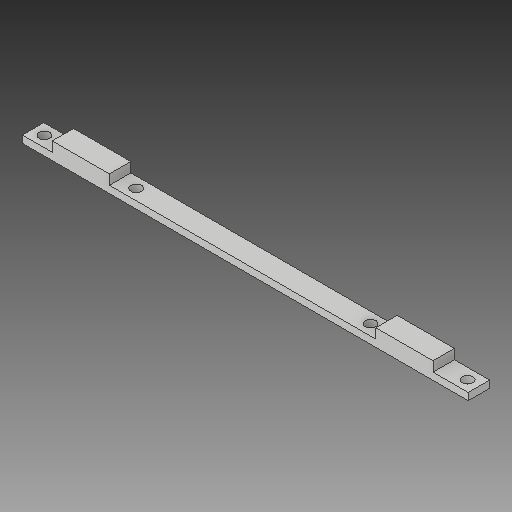
# Autodesk Inventor part: better support stick
Saved by Autodesk Inventor 2018 (Build 220112000, 112)
## iProperties
Created: 2019-09-14
Part Number: better support stick
Material: Generic
Document SubType Name: Modeling
Designer: Jacob
Density: 1 g/cm^3
Appearance: Default
Mass: 1.96771 g
Surface Area: 22.7987 cm^2
Volume: 1.96771 cm^3
Author: Jacob
Autodesk Inventor part; units mm, degrees
ref_plane "YZ Plane" through (0, 0, 0) normal (1, 0, 0) x (0, 1, 0)
ref_plane "XZ Plane" through (0, 0, 0) normal (0, 1, 0) x (-1, 0, 0)
ref_plane "XY Plane" through (0, 0, 0) normal (0, 0, 1) x (1, 0, 0)
sketch "Sketch1" plane through (0, 0, 0) normal (0, 1, 0) x (-1, 0, 0)
  line L0 (62.3443, -3) -> (-62.3443, -3)
  line L1 (-62.3443, -3) -> (-62.3443, 3)
  line L2 (-62.3443, 3) -> (62.3443, 3)
  line L3 (62.3443, 3) -> (62.3443, -3)
  line L4 (62.3443, -3) -> (-62.3443, 3) construction
  line L5 (-62.3443, -3) -> (62.3443, 3) construction
  line L6 (62.3443, 0) -> (-62.3443, 0) construction
  circle A0 centre (33.499, 0) radius 1.5
  circle A1 centre (-32.001, 0) radius 1.5
  line L7 (-55.499, -3) -> (-55.499, 3) construction
  line L8 (-55.499, 0) -> (-62.3443, 0) construction
  line L9 (52.501, -3) -> (52.501, 3) construction
  line L10 (62.3443, 0) -> (52.501, 0) construction
  line L11 (59.1693, -3) -> (59.1693, 3) construction
  line L12 (-59.1693, -3) -> (-59.1693, 3) construction
  circle A2 centre (-59.1693, 0) radius 1.5
  circle A3 centre (59.1693, 0) radius 1.5
  point P0 (0, 0)
  dimension "d0" = 65.5
  dimension "d1" = 3
  dimension "d2" = 3
  dimension "d3" = 6
  dimension "d7" = 3
  dimension "d8" = 3
  dimension "d17" = 124.6886
  dimension "d18" = 3.175
  dimension "d19" = 3.175
  constraints: 26 end point, 10 point on line, 8 midpoint, 4 centre point, 4 perpendicular, 2 parallel, 1 collinear, 1 horizontal, 1 vertical
  measures "d0" distance of A1.centre A0.centre
  measures "d1" diameter of A1
  measures "d2" diameter of A0
  measures "d3" distance of L0.end L1.end
  measures "d7" diameter of A2
  measures "d8" diameter of A3
  measures "d17" distance between parallel lines of L1 L3
  measures "d18" distance between parallel lines of L3 L11
  measures "d19" distance between parallel lines of L1 L12
extrude "Extrusion1" add sketch "Sketch1" along normal blind 2
sketch "Sketch2" plane through (0, 2, 0) normal (0, 1, 0) x (1, 0, 0)
  circle A0 centre (-33.499, 0) radius 1.5 projected
  line L0 (-33.499, 0) -> (-33.499, 3)
  line L1 (62.3443, 3) -> (-62.3443, 3) projected
  line L2 (-37.999, 0) -> (-37.999, 3)
  line L3 (-62.3443, -3) -> (62.3443, -3) projected
  line L4 (-37.999, 3) -> (-53.999, 3)
  line L5 (-53.999, 3) -> (-53.999, -3)
  line L6 (-53.999, -3) -> (-37.999, -3)
  line L7 (-37.999, -3) -> (-37.999, 3)
  line L8 (36.501, 3) -> (52.501, 3)
  line L9 (52.501, 3) -> (52.501, -3)
  line L10 (52.501, -3) -> (36.501, -3)
  line L11 (36.501, -3) -> (36.501, 3)
  circle A1 centre (32.001, 0) radius 1.5 projected
  point P0 (0, 0)
  dimension "d20" = 4.5
  dimension "d21" = 16
  dimension "d22" = 4.5
  dimension "d23" = 16
  constraints: 20 end point, 4 parallel, 4 point on line, 2 horizontal, 2 perpendicular, 2 vertical
  measures "d20" distance between parallel lines of L0 L2
  measures "d21" distance between parallel lines of L7 L5
  measures "d22" distance from line of A1.centre L11
  measures "d23" distance between parallel lines of L9 L11
extrude "Extrusion2" add sketch "Sketch2" along normal blind 2.75 contours L9 L3 L11 L1 | L2 L7 L3 L5 L1
fillet "Fillet1" [suppressed]
body "Solid1"
